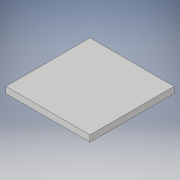
# Autodesk Inventor part: lowerbase
Saved by Autodesk Inventor 2019 (Build 230136000, 136)
## iProperties
Created: 2020-02-20
Part Number: lowerbase
Material: Generic
Document SubType Name: Modeling
Designer: ADMIN
Density: 1 g/cm^3
Appearance: Default
Author: ADMIN
Autodesk Inventor part; units mm, degrees
ref_plane "YZ Plane" through (0, 0, 0) normal (1, 0, 0) x (0, 1, 0)
ref_plane "XZ Plane" through (0, 0, 0) normal (0, 1, 0) x (-1, 0, 0)
ref_plane "XY Plane" through (0, 0, 0) normal (0, 0, 1) x (1, 0, 0)
sketch "Sketch1" plane through (0, 0, 0) normal (0, 1, 0) x (-1, 0, 0)
  line L0 (12.5529, 27.1991) -> (-387.4471, 27.1991)
  line L1 (-387.4471, 27.1991) -> (-387.4471, -372.8009)
  line L2 (-387.4471, -372.8009) -> (12.5529, -372.8009)
  line L3 (12.5529, -372.8009) -> (12.5529, 27.1991)
  point P0 (0, 0)
  dimension "d0" = 400
  dimension "d1" = 400
  dimension "d2" = 400
  constraints: 8 end point, 2 perpendicular, 1 horizontal
  measures "d0" distance of L0.start L0.end
  measures "d1" distance of L0.end L1.end
  measures "d2" distance of L1.end L2.end
extrude "Extrusion1" add sketch "Sketch1" along normal blind 30
body "Solid1"
